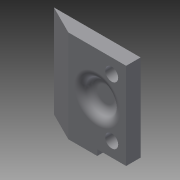
# Autodesk Inventor part: clip_tip
Saved by Autodesk Inventor 2015 (Build 190159000, 159)
## iProperties
Created: 2017-10-02
Part Number: clip_tip
Material: Generic
Document SubType Name: Modeling
Designer: Anshul
Density: 1 g/cm^3
Appearance: Default
Author: Anshul
Autodesk Inventor part; units mm, degrees
ref_plane "YZ Plane" through (0, 0, 0) normal (1, 0, 0) x (0, 1, 0)
ref_plane "XZ Plane" through (0, 0, 0) normal (0, 1, 0) x (-1, 0, 0)
sketch "Sketch1" plane through (0, 0, 0) normal (0, 1, 0) x (-1, 0, 0)
  line L0 (0, 0) -> (30, 0)
  line L1 (0, 5) -> (0, 0)
  line L2 (20, 5) -> (30, 0)
  line L3 (30, 12) -> (0, 12)
  line L4 (0, 12) -> (0, 5)
  line L5 (0, 5) -> (0, 7)
  line L6 (18, 7) -> (30, 12)
  line L7 (20, 5) -> (10, 5)
  line L8 (10, 5) -> (10, 7)
  line L9 (18, 7) -> (10, 7)
  line L10 (10, 5) -> (0, 5)
  line L11 (10, 5) -> (10, 0)
  dimension "d13" = 2
  dimension "d15" = 10
  constraints: 24 end point, 3 perpendicular, 3 point on line, 2 horizontal
  measures "d13" distance of L1.start L5.end
  measures "d15" distance of L2.start L7.end
extrude "Extrusion2" add sketch "Sketch1" along normal blind 30 contours L1 L10 L11 L0 | L11 L7 L2 L0
ref_plane "Work Plane2" through (-20, -2, 5) normal (0, 0, 1) x (1, 0, 0)
sketch "Sketch2" plane through (-20, -2, 5) normal (0, 0, 1) x (1, 0, 0)
  line L0 (20, 2) -> (20, 17)
  line L1 (20, 2) -> (20, 32) projected
  line L2 (20, 17) -> (10, 17)
  circle A0 centre (10, 17) radius 5
  circle A1 centre (10, 17) radius 7.5
  line L3 (20, 32) -> (15, 32)
  line L4 (20, 32) -> (-10, 32) projected
  line L5 (15, 32) -> (15, 27)
  circle A2 centre (15, 27) radius 2.25
  line L6 (20, 17) -> (20, 7)
  line L7 (20, 2) -> (20, 32) projected
  line L8 (20, 7) -> (15, 7)
  circle A3 centre (15, 7) radius 2.25
  dimension "d20" = 10
  dimension "d21" = 10
  dimension "d22" = 15
  dimension "d30" = 5
  dimension "d31" = 5
  dimension "d32" = 4.5
  dimension "d33" = 10
  dimension "d34" = 5
  dimension "d35" = 4.5
  constraints: 12 end point, 4 centre point, 4 coincident, 2 perpendicular, 2 point on line, 1 horizontal, 1 midpoint
  measures "d20" distance of L0.end L2.end
  measures "d21" diameter of A0
  measures "d22" diameter of A1
  measures "d30" distance of L1.end L3.end
  measures "d31" distance of L3.end L5.end
  measures "d32" diameter of A2
  measures "d33" distance of L0.end L6.end
  measures "d34" distance of L6.end L8.end
  measures "d35" diameter of A3
extrude "Extrusion3" cut sketch "Sketch2" against normal blind 3 contours A0
fillet "Fillet3" radius 3 2 edges at (-15, 15, 5) (-15, 15, 2)
extrude "Extrusion4" add sketch "Sketch1" against normal blind 2 contours L11 L7 L2 L0
extrude "Extrusion5" cut sketch "Sketch2" against normal blind 20 contours A2 | A3
body "Solid1"
